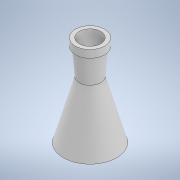
# Autodesk Inventor part: Модель колба коническая 25мл 1
Saved by Autodesk Inventor 2022 (Build 260153000, 153)
## iProperties
Created: 2022-06-09
Part Number: Модель колба коническая 25мл 1
Material: Типовые
Document SubType Name: Modeling
Designer: Admin
Density: 1 g/cm^3
Appearance: По умолчанию
Author: Admin
Autodesk Inventor part; units mm, degrees
ref_plane "YZ Plane" through (0, 0, 0) normal (1, 0, 0) x (0, 1, 0)
ref_plane "XZ Plane" through (0, 0, 0) normal (0, 1, 0) x (-1, 0, 0)
ref_plane "XY Plane" through (0, 0, 0) normal (0, 0, 1) x (1, 0, 0)
sketch "Эскиз1" plane through (0, 0, 0) normal (0, 0, 1) x (1, 0, 0)
  line L0 (0, 0) -> (21, 0)
  line L1 (21, 0) -> (8.5546, 45)
  line L2 (8.5546, 45) -> (10.0659, 65)
  line L3 (11.5, 65.5) -> (11.5, 71.5)
  line L4 (11.5, 71.5) -> (8.482, 71.5)
  line L5 (8.482, 71.5) -> (6.4795, 45)
  line L6 (6.4795, 45) -> (18.3718, 2)
  line L7 (18.3718, 2) -> (0, 2)
  line L8 (0, 21.2466) -> (0, -2.9394)
  line L9 (10.0659, 65) -> (11.5, 65.5)
  point P0 (0, 2)
  dimension "d1" = 2
  dimension "d2" = 2
  dimension "d13" = 21
  dimension "d14" = 12.959
  dimension "d15" = 16.964
  dimension "d16" = 11.5
  dimension "d17" = 0.5
  dimension "d18" = 6
  dimension "d19" = 20
  dimension "d20" = 45
  constraints: 20 end point, 3 parallel, 2 horizontal, 1 horizontal alignment, 1 perpendicular, 1 point on line, 1 vertical, 1 vertical alignment
  measures "d1" distance between parallel lines of L7 L0
  measures "d2" distance between parallel lines of L1 L6
  measures "d13" distance of L0.start L0.end
  measures "d14" diameter of L5.end L8
  measures "d15" diameter of L4.end L8
  measures "d16" distance from line of L0.start L3
  measures "d17" vertical distance of L3.start L2.end
  measures "d18" distance of L3.start L3.end
  measures "d19" vertical distance of L1.end L2.end
  measures "d20" vertical distance of L0.end L1.end
revolve "Вращение1" add sketch "Эскиз1" angle 360 about axis through (0, 21.2466, 0) along (0, -1, 0)
